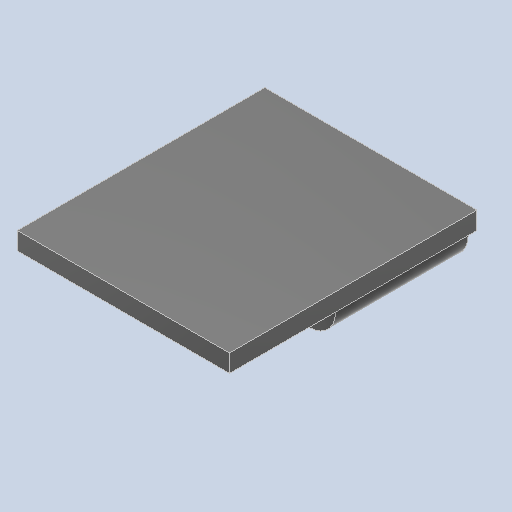
# Autodesk Inventor part: usb
Saved by Autodesk Inventor 2025.2 (Build 292293000, 293)
## iProperties
Created: 2024-04-03
Part Number: usb
Material: Acetal Resin, Black
Document SubType Name: Modeling
Designer: mirun
Density: 1.425 g/cm^3
Appearance: Smooth - Black
Author: mirun
Autodesk Inventor part; units mm, degrees
ref_plane "YZ Plane" through (0, 0, 0) normal (1, 0, 0) x (0, 1, 0)
ref_plane "XZ Plane" through (0, 0, 0) normal (0, 1, 0) x (-1, 0, 0)
ref_plane "XY Plane" through (0, 0, 0) normal (0, 0, 1) x (1, 0, 0)
sketch "Sketch1" plane through (0, 0, 0) normal (0, 0, 1) x (1, 0, 0)
  line L0 (-3, 0) -> (3, 0) construction
  line L1 (-3, -1.5) -> (3, -1.5)
  line L2 (3, 1.5) -> (-3, 1.5)
  arc A0 (-3, 1.5) -> (-3, -1.5) centre (-3, 0) ccw
  arc A1 (3, -1.5) -> (3, 1.5) centre (3, 0) ccw
  point P0 (0, 0)
  point P1 (4.5, 0)
  point P2 (-4.5, 0)
  dimension "d0" = 3
  dimension "d1" = 9
  constraints: 8 end point, 6 point on circle, 4 tangent, 2 centre point, 1 horizontal, 1 midpoint, 1 parallel
  measures "d0" diameter of A1
  measures "d1" distance of point (4.5, 0) point (-4.5, 0)
extrude "Extrusion1" add sketch "Sketch1" along normal blind 7.5
sketch "Sketch2" plane through (-3, 1.5, 0) normal (0, 1, 0) x (1, 0, 0)
  line L0 (6, 0) -> (0, 0) construction
  line L1 (9, -15) -> (-3, -15)
  line L2 (-3, -15) -> (-3, -1)
  line L3 (-3, -1) -> (9, -1)
  line L4 (9, -1) -> (9, -15)
  line L5 (9, -15) -> (-3, -1) construction
  line L6 (-3, -15) -> (9, -1) construction
  point P0 (3, 0)
  point P1 (3, -8)
  point P2 (3, 0)
  dimension "d4" = 1
  dimension "d5" = 12
  dimension "d6" = 14
  constraints: 12 end point, 3 midpoint, 2 parallel, 1 horizontal, 1 perpendicular, 1 vertical alignment
  measures "d4" distance between parallel lines of L3 L0
  measures "d5" distance between parallel lines of L4 L2
  measures "d6" distance between parallel lines of L1 L3
extrude "Extrusion2" add sketch "Sketch2" along normal blind 1
body "Solid1"
